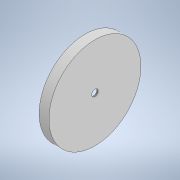
# Autodesk Inventor part: Housing_stage_close
Saved by Autodesk Inventor 2020 (Build 240168000, 168)
## iProperties
Created: 2020-05-12
Part Number: Housing_stage_close
Material: Generic
Document SubType Name: Modeling
Designer: avi41
Density: 1 g/cm^3
Appearance: Default
Author: avi41
Autodesk Inventor part; units mm, degrees
ref_plane "YZ Plane" through (0, 0, 0) normal (1, 0, 0) x (0, 1, 0)
ref_plane "XZ Plane" through (0, 0, 0) normal (0, 1, 0) x (-1, 0, 0)
ref_plane "XY Plane" through (0, 0, 0) normal (0, 0, 1) x (1, 0, 0)
sketch "Sketch1" plane through (0, 0, 0) normal (0, 1, 0) x (-1, 0, 0)
  line L0 (0, -86) -> (0, 8.5) construction
  line L1 (-4.1, 0) -> (17.6, 0) construction
  line L2 (-1, -5) -> (-1, -72.5)
  line L3 (-1, -72.5) -> (14.5, -72.5)
  line L4 (1, -5) -> (-1, -5)
  line L5 (14.5, -72.5) -> (14.5, -67.5)
  line L6 (1, -5) -> (1, -67.5)
  line L7 (1, -67.5) -> (14.5, -67.5)
  point P0 (1, -23.5)
  dimension "d7" = 5
  dimension "d28" = 5
  dimension "d29" = 2
  dimension "d30" = 13.5
  dimension "d31" = 72.5
  constraints: 12 end point, 3 perpendicular, 2 vertical, 1 point on line, 1 other
  measures "d7" distance between parallel lines of L1 L4
  measures "d28" distance between parallel lines of L3 L7
  measures "d29" distance between parallel lines of L2 L6
  measures "d30" distance between parallel lines of L6 L5
  measures "d31" distance between parallel lines of L1 L3
revolve "Revolution1" add sketch "Sketch1" angle 360 about axis through (0, 0, 0) along (-1, 0, 0)
equation "\"D_ring\" = D_ext"
equation "\"D_ext\" = 139.15534"
body "Solid1"
